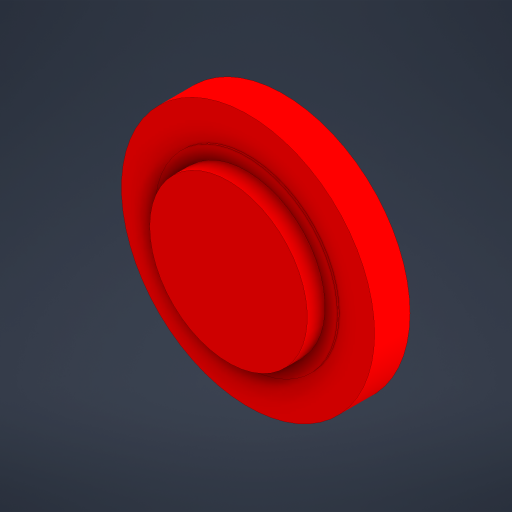
# Autodesk Inventor part: Outer Ring Press
Saved by Autodesk Inventor 2023.4 (Build 274418000, 418)
## iProperties
Created: 2024-07-23
Part Number: Outer Ring Press
Material: Generic
Document SubType Name: Modeling
Designer: xSibe
Density: 1 g/cm^3
Appearance: Plastic Red
Author: xSibe
Autodesk Inventor part; units mm, degrees
ref_plane "YZ Plane" through (0, 0, 0) normal (1, 0, 0) x (0, 1, 0)
ref_plane "XZ Plane" through (0, 0, 0) normal (0, 1, 0) x (-1, 0, 0)
ref_plane "XY Plane" through (0, 0, 0) normal (0, 0, 1) x (1, 0, 0)
sketch "Sketch1" plane through (0, 0, 0) normal (0, 0, 1) x (1, 0, 0)
  circle A0 centre (0, 0) radius 11.125
  circle A1 centre (0, 0) radius 12.875
  circle A2 centre (0, 0) radius 17.875
  dimension "d0" = 22.25
  dimension "d1" = 25.75
  dimension "d2" = 5
  constraints: 3 centre point, 2 coincident
  measures "d0" diameter of A0
  measures "d1" diameter of A1
  measures "d2" radial gap between concentric circles of A1 A2
extrude "Extrusion1" add sketch "Sketch1" along normal blind 5 contours A0 | A1 | A2
extrude "Extrusion2" add sketch "Sketch1" along normal blind 0.25 from surface at 5 contours A0 | A1
extrude "Extrusion3" add sketch "Sketch1" along normal blind 2.5 from surface at 5.25 contours A0
body "Solid1"
